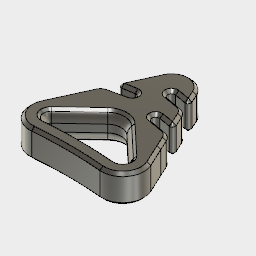
GuylineQuickAdjusterV4 (Autodesk Fusion 360 design; units mm, degrees)
Autodesk Fusion 360 part; units mm, degrees
sketch "Sketch1" plane through (0, 0, 0) normal (0, 0, 1) x (1, 0, 0)
  line L0 (6.8858, 1.5185) -> (1.7078, 6.3879)
  line L1 (8.5, 0) -> (18.6301, 0) construction
  line L2 (-6.8872, 1.5179) -> (-1.719, 6.3864)
  arc A0 (6.3068, 0.2249) -> (-6.3077, 0.2249) centre (-0.0001, -72) ccw
  arc A1 (-6.8872, 1.5179) -> (-6.3077, 0.2249) centre (-6.3729, 0.972) ccw
  arc A2 (6.3068, 0.2249) -> (6.8858, 1.5185) centre (6.372, 0.9721) ccw
  arc A3 (1.7078, 6.3879) -> (-1.719, 6.3864) centre (-0.0048, 4.5667) ccw
  arc A4 (-9.7878, 2.5199) -> (-6.0467, -2.7631) centre (-6.3729, 0.972) ccw
  arc A5 (6.0459, -2.763) -> (-6.0467, -2.7631) centre (-0.0001, -72) ccw
  arc A6 (6.0459, -2.763) -> (9.7871, 2.5196) centre (6.372, 0.9721) ccw
  line L3 (-0.0059, 7.0667) -> (-0.006, 7.5)
  line L4 (-0.0059, 7.0667) -> (-0.0183, 10.5002) construction
  line L5 (-0.0183, 10.5002) -> (-0.0001, 12.0001) construction
  line L6 (-0.0001, 12.0001) -> (0.0118, 15.0001) construction
  line L7 (0.0118, 15.0001) -> (6.9877, 13.7494) construction
  line L8 (-0.0183, 10.5002) -> (11.6288, 8.4465) construction
  line L9 (-0.0183, 10.5002) -> (11.5483, 10.5002) construction
  line L10 (-0.0001, 12.0001) -> (-12.6146, 9.7758) construction
  line L11 (-0.0001, 12.0001) -> (12.8092, 12.0001) construction
  line L12 (-4.6694, 11.8388) -> (-2.6197, 12.1977)
  line L13 (-2.3973, 10.9169) -> (-5.3701, 10.2906)
  line L14 (-6.7795, 9.159) -> (-9.7878, 2.5199)
  line L15 (8.2335, 5.8598) -> (9.7871, 2.5196)
  line L16 (-0.0945, 14.4622) -> (0.0357, 14.4389)
  line L17 (0.937, 14.2773) -> (3.6482, 13.7912)
  arc A7 (-2.3973, 10.9169) -> (-2.6197, 12.1977) centre (-2.5076, 11.5574) ccw
  arc A8 (-5.2114, 12.5369) -> (-4.6694, 11.8388) centre (-4.7556, 12.3313) ccw
  arc A9 (-5.3701, 10.2906) -> (-6.7795, 9.159) centre (-4.9578, 8.3335) ccw
  arc A10 (5.1129, 12.6571) -> (3.6482, 13.7912) centre (3.2953, 11.8226) ccw
  line L18 (5.3735, 10.2095) -> (3.3582, 10.5649)
  line L19 (5.1129, 12.6571) -> (5.9147, 10.9105)
  line L20 (7.4094, 7.6548) -> (8.2335, 5.8598)
  line L21 (3.1495, 9.2819) -> (5.9391, 8.79)
  arc A11 (3.3582, 10.5649) -> (3.1495, 9.2819) centre (3.2453, 9.9248) ccw
  arc A12 (5.3735, 10.2095) -> (5.9147, 10.9105) centre (5.4603, 10.7019) ccw
  arc A13 (7.4094, 7.6548) -> (5.9391, 8.79) centre (5.5918, 6.8204) ccw
  line L22 (3.1691, 15.2021) -> (1.1684, 15.5547)
  arc A14 (1.1684, 15.5547) -> (0.9892, 14.2679) centre (1.0556, 14.9145) ccw
  line L23 (3.7111, 15.9013) -> (3.0429, 17.3727)
  line L24 (-5.2114, 12.5369) -> (-3.0057, 17.3767)
  arc A15 (3.0429, 17.3727) -> (-3.0057, 17.3767) centre (0.0177, 15.9989) ccw
  arc A16 (3.1691, 15.2021) -> (3.7111, 15.9013) centre (3.2559, 15.6945) ccw
  line L25 (0.1442, 15.7383) -> (7.1201, 14.4876) construction
  point P0 (-5.5748, 11.6802)
  point P1 (7.0718, 8.5146)
  point P2 (6.3126, 10.0439)
  dimension "d4" = 0.75
  dimension "d5" = 0.75
  dimension "d6" = 2.5
  dimension "d13" = 1.5
  dimension "d14" = 3
  dimension "d16" = 10
  dimension "d17" = 170
  dimension "d24" = 3
  dimension "d30" = 0.5
  dimension "d31" = 2
  dimension "d33" = 2
  dimension "d41" = 3
  dimension "d42" = 0.5
  dimension "d43" = 2
  dimension "d44" = 0.75
  dimension "d45" = 0.5
  dimension "d52" = 0.65
  dimension "d53" = 0.65
  dimension "d54" = 0.65
  measures "d4" radius of A1
  measures "d5" radius of A2
  measures "d6" radius of A3
  measures "d13" distance of L4.end L5.end
  measures "d14" distance of L5.end L6.end
  measures "d16" angle of L8 L9
  measures "d17" angle of L10 L11
  measures "d24" distance of P0 L12.end
  measures "d30" radius of A8
  measures "d31" radius of A9
  measures "d33" radius of A10
  measures "d41" distance of P2 L18.end
  measures "d42" radius of A12
  measures "d43" radius of A13
  measures "d45" radius of A16
  measures "d52" radius of A14
  measures "d53" radius of A7
  measures "d54" radius of A11
extrude "Extrude1" add sketch "Sketch1" along normal blind 5
chamfer "Chamfer1" distance 0.5 angle 45 50 edges at (-3.8837, 10.6037, 5) (-6.2099, 9.8931, 5) (-8.2836, 5.8394, 5) (-9.4327, -1.1947, 5) (-0.0004, -2.4995, 5) (9.4317, -1.1948, 5) (9.0103, 4.1897, 5) (7.8214, 6.7573, 5) (6.814, 8.4034, 5) (4.5443, 9.0359, 5) (-3.8837, 10.6037, 0) (-6.2099, 9.8931, 0) (-8.2836, 5.8394, 0) (-9.4327, -1.1947, 0) (-0.0004, -2.4995, 0) (9.4317, -1.1948, 0) (9.0103, 4.1897, 0) (7.8214, 6.7573, 0) (6.814, 8.4034, 0) (4.5443, 9.0359, 0) (2.6037, 10.0291, 5) (4.3658, 10.3872, 5) (5.8561, 10.3964, 5) (5.5138, 11.7838, 5) (4.5198, 13.4039, 5) (2.3187, 14.0296, 5) (0.4118, 15.0042, 5) (2.1687, 15.3784, 5) (3.651, 15.3882, 5) (3.377, 16.637, 5) (0.0199, 19.3214, 5) (-4.1086, 14.9568, 5) (-5.1506, 12.0246, 5) (-3.6445, 12.0182, 5) (-1.8672, 11.6687, 5) (2.3187, 14.0296, 0) (4.5198, 13.4039, 0) (5.5138, 11.7838, 0) (5.8561, 10.3964, 0) (4.3658, 10.3872, 0) (2.6037, 10.0291, 0) (-1.8672, 11.6687, 0) (-3.6445, 12.0182, 0) (-5.1506, 12.0246, 0) (-4.1086, 14.9568, 0) (0.0199, 19.3214, 0) (3.377, 16.637, 0) (3.651, 15.3882, 0) (2.1687, 15.3784, 0) (0.4118, 15.0042, 0)
chamfer "Chamfer2" distance 1 angle 45 6 edges at (7.0566, 0.6657, 5) (-0.0004, 0.4998, 5) (-7.0573, 0.6653, 5) (-4.3031, 3.9522, 5) (-0.0059, 7.0667, 5) (4.2968, 3.9532, 5)
chamfer "Chamfer3" distance 1 angle 45 6 edges at (7.0566, 0.6657, 0) (-0.0004, 0.4998, 0) (-7.0573, 0.6653, 0) (-4.3031, 3.9522, 0) (-0.0059, 7.0667, 0) (4.2968, 3.9532, 0)
fillet "Fillet1" radius 2 12 edges at (7.0566, 0.6657, 4) (-0.0004, 0.4998, 4) (-7.0573, 0.6653, 4) (-4.3031, 3.9522, 4) (-0.0059, 7.0667, 4) (4.2968, 3.9532, 4) (-7.0573, 0.6653, 1) (-0.0004, 0.4998, 1) (7.0566, 0.6657, 1) (4.2968, 3.9532, 1) (-0.0059, 7.0667, 1) (-4.3031, 3.9522, 1)
